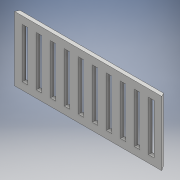
# Autodesk Inventor part: pcbcover
Saved by Autodesk Inventor 2017 (Build 210142000, 142)
## iProperties
Created: 2017-08-24
Part Number: pcbcover
Material: Generic
Document SubType Name: Modeling
Designer: erwin
Density: 1 g/cm^3
Appearance: Default
Author: erwin
Autodesk Inventor part; units mm, degrees
ref_plane "YZ Plane" through (0, 0, 0) normal (1, 0, 0) x (0, 1, 0)
ref_plane "XZ Plane" through (0, 0, 0) normal (0, 1, 0) x (-1, 0, 0)
ref_plane "XY Plane" through (0, 0, 0) normal (0, 0, 1) x (1, 0, 0)
sketch "Sketch1" plane through (0, 0, 0) normal (0, 1, 0) x (-1, 0, 0)
  line L0 (0, 0) -> (-3, 0)
  line L1 (-3, 0) -> (-3, -27)
  line L2 (-3, -27) -> (0, -27)
  line L3 (0, -27) -> (0, 0)
  line L4 (-7.62, 0) -> (-10.62, 0)
  line L5 (-10.62, 0) -> (-10.62, -27)
  line L6 (-10.62, -27) -> (-7.62, -27)
  line L7 (-7.62, -27) -> (-7.62, 0)
  line L8 (-15.24, 0) -> (-18.24, 0)
  line L9 (-18.24, 0) -> (-18.24, -27)
  line L10 (-18.24, -27) -> (-15.24, -27)
  line L11 (-15.24, -27) -> (-15.24, 0)
  line L12 (-22.86, 0) -> (-25.86, 0)
  line L13 (-25.86, 0) -> (-25.86, -27)
  line L14 (-25.86, -27) -> (-22.86, -27)
  line L15 (-22.86, -27) -> (-22.86, 0)
  line L16 (-30.48, 0) -> (-33.48, 0)
  line L17 (-33.48, 0) -> (-33.48, -27)
  line L18 (-33.48, -27) -> (-30.48, -27)
  line L19 (-30.48, -27) -> (-30.48, 0)
  line L20 (-38.1, 0) -> (-41.1, 0)
  line L21 (-41.1, 0) -> (-41.1, -27)
  line L22 (-41.1, -27) -> (-38.1, -27)
  line L23 (-38.1, -27) -> (-38.1, 0)
  line L24 (-45.72, 0) -> (-48.72, 0)
  line L25 (-48.72, 0) -> (-48.72, -27)
  line L26 (-48.72, -27) -> (-45.72, -27)
  line L27 (-45.72, -27) -> (-45.72, 0)
  line L28 (-53.34, 0) -> (-56.34, 0)
  line L29 (-56.34, 0) -> (-56.34, -27)
  line L30 (-56.34, -27) -> (-53.34, -27)
  line L31 (-53.34, -27) -> (-53.34, 0)
  line L32 (-60.96, 0) -> (-63.96, 0)
  line L33 (-63.96, 0) -> (-63.96, -27)
  line L34 (-63.96, -27) -> (-60.96, -27)
  line L35 (-60.96, -27) -> (-60.96, 0)
  line L36 (-68.58, 0) -> (-71.58, 0)
  line L37 (-71.58, 0) -> (-71.58, -27)
  line L38 (-71.58, -27) -> (-68.58, -27)
  line L39 (-68.58, -27) -> (-68.58, 0)
  line L40 (0, 0) -> (-71.58, 0) construction
  line L41 (-71.58, 0) -> (-71.58, -27) construction
  line L42 (-71.58, -27) -> (0, -27) construction
  line L43 (0, -27) -> (0, 0) construction
  line L44 (-75.79, 4) -> (4.21, 4)
  line L45 (4.21, 4) -> (4.21, -31)
  line L46 (4.21, -31) -> (-75.79, -31)
  line L47 (-75.79, -31) -> (-75.79, 4)
  line L48 (-75.79, 4) -> (4.21, -31) construction
  line L49 (4.21, 4) -> (-75.79, -31) construction
  point P0 (-35.79, -13.5)
  dimension "d0" = 3
  dimension "d1" = 27
  dimension "d4" = 7.62
  dimension "d9" = 80
  dimension "d10" = 35
  constraints: 100 end point, 6 parallel, 4 horizontal, 3 perpendicular, 2 midpoint, 1 collinear, 71 other
  measures "d0" distance of L2.end L1.end
  measures "d1" distance of L1.end L0.end
  measures "d4" distance of L0.start L4.start
  measures "d9" distance of L45.end L46.end
  measures "d10" distance of L44.end L45.end
extrude "Extrusion1" add sketch "Sketch1" along normal blind 2
chamfer "Chamfer1" distance 1 distance2 2 1 edges at (-4.21, 2, -13.5) measured on face at (36.56, 2, -29.6667)
chamfer "Chamfer2" distance 1 distance2 2 1 edges at (36.2897, 2, -31) measured on face at (36.8932, 2, -29.6667)
chamfer "Chamfer3" distance 1 distance2 2 1 edges at (75.79, 2, -13.0002) measured on face at (30.2732, 2, 2.6667)
body "Solid1"
